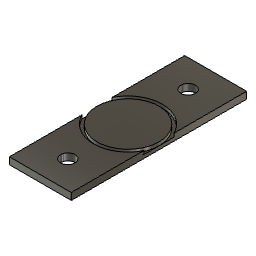
AnyBio_Piston_Bottom v3 (Autodesk Fusion 360 design; units mm, degrees)
Autodesk Fusion 360 part; units mm, degrees
note: some values were not read from the file. Set by a fixed rule: which sketch regions a step uses.
sketch "Sketch2" plane through (0, 0, 0) normal (0, 0, 1) x (1, 0, 0)
  line L0 (9, -25.5) -> (-9, -25.5)
  line L1 (-9, -25.5) -> (-9, 25.5)
  line L2 (-9, 25.5) -> (9, 25.5)
  line L3 (9, 25.5) -> (9, -25.5)
  line L4 (9, -25.5) -> (-9, 25.5) construction
  line L5 (-9, -25.5) -> (9, 25.5) construction
  line L6 (0, -25.5) -> (0, -17.5) construction
  line L7 (0, 25.5) -> (0, 17.5) construction
  circle A0 centre (0, 17.5) radius 2.1
  circle A1 centre (0, -17.5) radius 2.1
  dimension "d17" = 18
  dimension "d18" = 51
  dimension "d19" = 8
  dimension "d20" = 8
  dimension "d21" = 4.2
  dimension "d22" = 4.2
  constraint horizontal L0
  constraint perpendicular L0 L1
  constraint parallel L0 L2
  constraint parallel L1 L3
  constraint coincident L4 origin
  constraint coincident L5 origin
  constraint midpoint L0 L6.start
  constraint perpendicular L0 L6
  constraint vertical L7
  constraint midpoint L2 L7.start
  constraint coincident L7.end A0.centre
  constraint coincident L6.end A1.centre
  measures "d17" distance of L1.end L2.end
  measures "d18" distance of L0.end L1.end
  measures "d19" distance of L6.start L6.end
  measures "d20" distance of L7.start L7.end
  measures "d21" diameter of A0
  measures "d22" diameter of A1
extrude "Extrude3" add sketch "Sketch2" along normal blind 2
sketch "Sketch3" plane through (0, 0, 2) normal (0, 0, 1) x (-1, 0, 0)
  circle A0 centre (0, -17.5) radius 2.1
  circle A1 centre (0, 17.5) radius 2.1
  line L0 (-9, -25.5) -> (9, -25.5)
  line L1 (9, -25.5) -> (9, 25.5)
  line L2 (9, 25.5) -> (-9, 25.5)
  line L3 (-9, 25.5) -> (-9, -25.5)
  circle A2 centre (0, 0) radius 9
  dimension "d25" = 18
  constraint coincident A2.centre origin
  measures "d25" diameter of A2
sketch "Sketch4" plane through (0, 0, 2) normal (0, 0, 1) x (-1, 0, 0)
  line L0 (-9, 25.5) -> (-9, -25.5)
  line L1 (-9, -25.5) -> (9, -25.5)
  line L2 (9, -25.5) -> (9, 25.5)
  circle A0 centre (0, -17.5) radius 2.1
  circle A1 centre (0, 0) radius 9
  circle A2 centre (0, 0) radius 10
  circle A3 centre (0, 17.5) radius 2.1
  line L3 (9, 25.5) -> (-9, 25.5)
  dimension "d28" = 20
  constraint coincident A1.centre A2.centre
  constraint concentric A1 A2
  measures "d28" diameter of A2
extrude "Extrude5" cut sketch "Sketch4" against normal blind 1 contours L0 L2 A1 A2 | L0 A2 | L0 L2 A1 A2 | L2 A2
named bodies: "Piston_Bottom"
